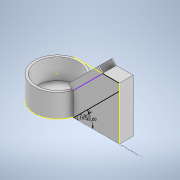
# Autodesk Inventor part: inclined container
Saved by Autodesk Inventor 2020.2 (Build 242310000, 310)
## iProperties
Created: 2020-03-03
Part Number: inclined container
Material: Generic
Document SubType Name: Modeling
Designer: Ajeya
Density: 1 g/cm^3
Appearance: Default
Author: Ajeya
Autodesk Inventor part; units mm, degrees
ref_plane "YZ Plane" through (0, 0, 0) normal (1, 0, 0) x (0, 1, 0)
ref_plane "XZ Plane" through (0, 0, 0) normal (0, 1, 0) x (-1, 0, 0)
ref_plane "XY Plane" through (0, 0, 0) normal (0, 0, 1) x (1, 0, 0)
sketch "Sketch1" plane through (0, 0, 0) normal (0, 1, 0) x (-1, 0, 0)
  circle A0 centre (0, 0) radius 100
  dimension "d0" = 100
  constraints: 1 centre point, 1 coincident
  measures "d0" radius of A0
extrude "Extrusion1" add sketch "Sketch1" along normal blind 100
sketch "Sketch2" plane through (0, 100, 0) normal (0, 1, 0) x (1, 0, 0)
  circle A0 centre (0, 0) radius 90
  dimension "d3" = 90
  constraints: 1 centre point, 1 coincident
  measures "d3" radius of A0
extrude "Extrusion2" cut sketch "Sketch2" against normal blind 90
sketch "Sketch3" plane through (0, 100, 0) normal (0, 1, 0) x (1, 0, 0)
  point P0 (0, 0)
sketch "Sketch4" plane through (0, 0, 0) normal (0, 0, 1) x (1, 0, 0)
  line L0 (100, 0) -> (100, 100) projected
  line L1 (100, 0) -> (-100, 0) projected
  line L2 (100, 100) -> (100, 0)
  point P0 (0, 0)
  constraints: 2 end point, 1 point on line, 1 vertical
sketch "Sketch5" plane through (0, 0, 0) normal (0, 1, 0) x (-1, 0, 0)
  circle A0 centre (0, 0) radius 100 projected
  line L0 (-95.5, 30.3394) -> (-95.5, 30.3394)
  circle A1 centre (0, 0) radius 100 projected
  line L1 (-100, 0) -> (-100, 30)
  line L2 (-100, 30) -> (-100, -30)
  dimension "d12" = 30
  dimension "d13" = 60
  constraints: 6 end point, 2 vertical, 1 horizontal alignment, 1 point on line, 1 other
  measures "d12" distance of L1.start L1.end
  measures "d13" distance of L1.end L2.end
sketch "Sketch6" plane through (0, 0, 0) normal (1, 0, 0) x (0, 1, 0)
  point P0 (0, 0)
sketch "Sketch7" plane through (0, 0, 0) normal (1, 0, 0) x (0, 1, 0)
  point P0 (0, 0)
sketch "Sketch8" plane through (0, 0, 0) normal (0, 0, 1) x (1, 0, 0)
  line L0 (71.0018, -29.5169) -> (371.0018, -29.5169) construction
  point P0 (0, 0)
  constraints: 2 end point, 1 horizontal
sketch "Sketch9" plane through (0, 0, 0) normal (1, 0, 0) x (0, 1, 0)
  point P0 (0, 0)
sketch "Sketch10" plane through (0, 0, 0) normal (1, 0, 0) x (0, 1, 0)
  point P0 (0, 0)
sketch "Sketch11" plane through (0, 100, 0) normal (0, 1, 0) x (1, 0, 0)
  point P0 (0, 0)
sketch "Sketch12" plane through (0, 0, 0) normal (0, 1, 0) x (-1, 0, 0)
  line L0 (-100, -28.9567) -> (-300, -28.9567)
  line L1 (-300, -28.9567) -> (-300, 31.0433)
  line L2 (-300, 31.0433) -> (-100, 31.0433)
  line L3 (-100, 31.0433) -> (-100, -28.9567)
  point P0 (0, 0)
  dimension "d16" = 200
  dimension "d17" = 60
  constraints: 8 end point, 2 parallel, 1 horizontal, 1 perpendicular
  measures "d16" distance of L1.end L2.end
  measures "d17" distance of L0.end L1.end
extrude "Extrusion3" add sketch "Sketch12" along normal blind 230
sketch "Sketch13" plane through (100, 0, 31.0433) normal (0, 0, 1) x (1, 0, 0)
  line L0 (0, 0) -> (-200, 0) projected
  line L1 (0, 0) -> (200, 200)
  line L2 (200, 0) -> (200, 230) projected
  line L3 (0, 0) -> (282.8427, 0) construction
  line L4 (0, 103.2812) -> (126.7188, 230)
  line L5 (0, 230) -> (200, 230) projected
  line L6 (126.7188, 230) -> (200, 230)
  line L7 (200, 200) -> (0, 0)
  line L8 (0, 103.2812) -> (126.7188, 230)
  point P0 (-100, 0)
  dimension "d20" = 45
  constraints: 12 end point, 2 point on line, 1 collinear, 1 equal length, 1 horizontal
  measures "d20" angle of L3 L1
chamfer "Chamfer1" distance 127 angle 45 1 edges at (100, 230, 1.0433)
sketch "Sketch14" plane through (227, 230, -28.9567) normal (-0.7071, 0.7071, 0) x (-0.7071, -0.7071, 0)
  line L0 (0, 0) -> (179.6051, 0) projected
  line L1 (179.6051, 0) -> (179.6051, 60) projected
  line L2 (0, 0) -> (179.6051, 0)
  line L3 (179.6051, 0) -> (179.6051, 5)
  line L4 (179.6051, 5) -> (0, 5)
  line L5 (0, 5) -> (0, 0)
  line L6 (0, 60) -> (0, 0) projected
  ellipse E0 centre (252.4371, 28.9567) end of major axis (252.4371, 128.9567) minor radius 70.7107 projected
  line L7 (0, 60) -> (184.1665, 60)
  line L8 (184.1665, 60) -> (184.1665, 55)
  line L9 (184.1665, 55) -> (0, 55)
  line L10 (0, 55) -> (0, 60)
  point P0 (323.1478, 28.9567)
  point P1 (181.7264, 28.9567)
  point P2 (0, 55)
  dimension "d24" = 5
  dimension "d25" = 5
  constraints: 16 end point, 4 parallel, 2 horizontal, 2 perpendicular, 1 point on line, 2 other
  measures "d24" distance of L3.end L2.end
  measures "d25" distance of L7.end L8.end
extrude "Extrusion4" add sketch "Sketch14" along normal blind 25.4 contours L6 L7 L1 L9 | L1 L7 L8 L9
sketch "Sketch15" plane through (227, 230, -28.9567) normal (-0.7071, 0.7071, 0) x (-0.7071, -0.7071, 0)
  line L0 (-51.6188, 0) -> (0, 0) projected
  line L1 (179.6051, 0) -> (179.6051, 55) projected
  line L2 (0, 0) -> (179.6051, 0)
  line L3 (179.6051, 0) -> (179.6051, 5)
  line L4 (179.6051, 5) -> (0, 5)
  line L5 (0, 5) -> (0, 0)
  point P0 (323.1478, 28.9567)
  point P1 (179.6051, 0)
  dimension "d28" = 5
  constraints: 8 end point, 2 parallel, 1 horizontal, 1 perpendicular, 1 point on line
  measures "d28" distance of L3.end L2.end
extrude "Extrusion5" add sketch "Sketch15" along normal blind 25.4
body "Solid1"
